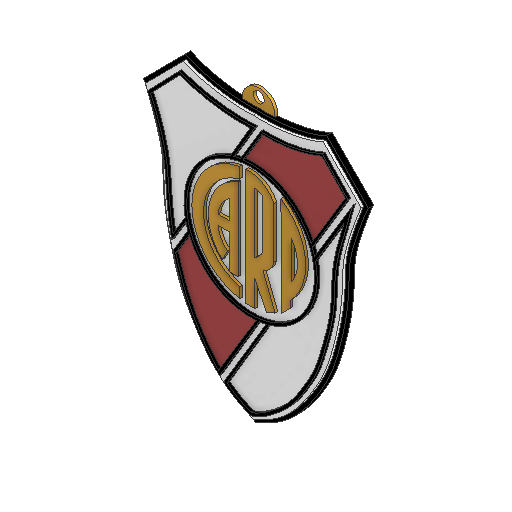
# Autodesk Inventor part: Sports Team Keychain
Saved by Autodesk Inventor 2026.2 (Build 302298000, 298)
## iProperties
Created: 2025-12-23
Part Number: Sports Team Keychain
Material: Generic
Document SubType Name: Modeling
Designer: andyeske
Density: 1 g/cm^3
Appearance: Default
Author: andyeske
Autodesk Inventor part; units mm, degrees
ref_plane "YZ Plane" through (0, 0, 0) normal (1, 0, 0) x (0, 1, 0)
ref_plane "XZ Plane" through (0, 0, 0) normal (0, 1, 0) x (-1, 0, 0)
ref_plane "XY Plane" through (0, 0, 0) normal (0, 0, 1) x (1, 0, 0)
sketch "Sketch1" plane through (0, 0, 0) normal (0, 0, 1) x (1, 0, 0)
  line L0 (-132.0665, 124.8918) -> (132.5169, 124.8918) construction
  line L1 (132.5169, 124.8918) -> (132.5169, -139.6916) construction
  line L2 (132.5169, -139.6916) -> (-132.0665, -139.6916) construction
  line L3 (-132.0665, -139.6916) -> (-132.0665, 124.8918) construction
  line L4 (0.2252, 52.8739) -> (0.2252, -73.7577) construction
  spline S0 degree 3 poles (0.2252, 52.8739) (-7.1403, 52.2049) (-23.4624, 53.7737) (-32.7052, 58.8275) knots 0 0 0 0 1 1 1 1
  line L5 (-32.7052, 58.8275) -> (-52.252, 39.1099)
  spline S1 degree 4 poles (-52.252, 39.1099) (-50.7995, 37.3406) (-43.3506, 15.7132) (-43.2795, 13.9138) (-43.0599, -7.6539) (-38.1267, -26.9843) (-33.574, -42.7818) (-15.201, -69.3664) (-7.1707, -69.2086) (0.2252, -73.7577) knots 0 0 0 0 0 0.249108 0.356574 0.465638 0.590869 0.717378 1 1 1 1 1
  spline S2 degree 3 poles (0.2252, 52.8739) (7.5907, 52.2049) (23.9128, 53.7737) (33.1557, 58.8275) knots 0 0 0 0 1 1 1 1
  line L6 (33.1557, 58.8275) -> (52.7024, 39.1099)
  spline S3 degree 4 poles (52.7024, 39.1099) (51.2499, 37.3406) (43.801, 15.7132) (43.7299, 13.9138) (43.5103, -7.6539) (38.5771, -26.9843) (34.0244, -42.7818) (15.6514, -69.3664) (7.6211, -69.2086) (0.2252, -73.7577) knots 0 0 0 0 0 0.249108 0.356574 0.465638 0.590869 0.717378 1 1 1 1 1
  line L7 (50.2121, 38.7692) -> (32.7643, 56.3696)
  line L8 (32.8267, 56.7373) -> (50.5783, 38.8306)
  line L9 (-50.1278, 38.8306) -> (-32.3763, 56.7373)
  circle A0 centre (0.2252, 1.113) radius 31.0921
  circle A1 centre (0.2252, 1.113) radius 29.8304
  arc A2 (-4.9144, 28.5122) -> (-4.8155, -24.875) centre (-0.0222, 1.8276) ccw
  arc A3 (-4.9144, 23.4163) -> (-4.8155, -20.0306) centre (0.7097, 1.7055) ccw
  arc A4 (-5.5588, 21.892) -> (-12.9917, -13.1761) centre (1.5498, 2.0635) ccw
  arc A5 (-9.6705, 13.2195) -> (-14.9692, 4.2431) centre (-2.5392, 2.9579) ccw
  arc A6 (-14.9692, -0.3288) -> (-10.4952, -8.5226) centre (-2.4753, 1.1746) ccw
  line L10 (-14.9692, -0.3288) -> (-9.6705, -0.3288)
  line L11 (-9.6705, -0.3288) -> (-9.6705, -16.3707)
  line L12 (-9.6705, -16.3707) -> (-5.5588, -16.3707)
  line L13 (-5.5588, -16.3707) -> (-5.5588, 21.892)
  line L14 (-9.6705, 13.2195) -> (-9.6705, 4.2431)
  line L15 (-9.6705, 4.2431) -> (-14.9692, 4.2431)
  line L16 (-10.4952, -8.5226) -> (-12.9917, -13.1761)
  line L17 (-4.8155, -20.0306) -> (-4.8155, -24.875)
  line L18 (-4.9144, 28.5122) -> (-4.9144, 23.4163)
  line L19 (-2.0198, 28.8256) -> (-2.0198, -25.345)
  line L20 (-2.0198, -25.345) -> (2.2612, -25.345)
  line L21 (2.2612, -25.345) -> (2.2612, -13.1046)
  line L22 (2.2612, -13.1046) -> (7.5833, -24.2139)
  line L23 (7.5833, -24.2139) -> (11.6912, -22.4528)
  line L24 (11.6912, -22.4528) -> (5.9834, -8.1423)
  line L25 (18.7175, -13.8348) -> (18.7175, -16.995)
  line L26 (18.7175, -16.995) -> (14.6967, -21.051)
  line L27 (14.6967, -21.051) -> (14.3943, 25.0785)
  line L28 (19.2337, -6.0507) -> (19.2337, 11.4074)
  line L29 (2.2612, 23.4163) -> (2.2612, -4.7023)
  line L30 (5.9834, -0.3288) -> (5.9834, 21.892)
  line L31 (11.1353, 21.5624) -> (11.1353, -2.0971)
  arc A7 (5.9834, 21.892) -> (2.2612, 23.4163) centre (1.1977, 15.5123) ccw
  arc A8 (11.1353, 21.5624) -> (-2.0198, 28.8256) centre (-0.5221, 15.9934) ccw
  arc A9 (2.2612, -4.7023) -> (5.9834, -0.3288) centre (-1.54, 2.3034) ccw
  arc A10 (5.9834, -8.1423) -> (11.1353, -2.0971) centre (2.8946, -0.2921) ccw
  arc A11 (19.2337, -6.0507) -> (19.2337, 11.4074) centre (7.6722, 2.6784) ccw
  arc A12 (18.7175, -13.8348) -> (14.3943, 25.0785) centre (0.6922, 3.8595) ccw
  arc A13 (-33.199, 52.8738) -> (2.2612, 47.7839) centre (-3.3286, 134.908) ccw
  line L32 (-33.199, 52.8738) -> (-47.9375, 37.5085)
  spline S4 degree 4 poles (-47.9375, 37.5085) (-46.8652, 36.0211) (-37.463, 13.2639) (-40.1687, 6.2328) (-38.1633, -9.6174) (-36.5654, -16.995) knots 0 0 0 0 0 0.485566 1 1 1 1 1
  line L33 (-46.4307, 37.3236) -> (-32.8677, 51.4634)
  arc A14 (-32.8677, 51.4634) -> (0, 46.4519) centre (-3.3286, 134.908) ccw
  line L34 (-35.9295, -14.0185) -> (-30.2885, -4.8559)
  line L35 (-36.5654, -16.995) -> (-29.9733, -6.2874)
  line L36 (2.2612, 47.7839) -> (-7.614, 31.2006)
  line L37 (-9.2032, 30.7411) -> (0, 46.4519)
  arc A15 (4.9226, 47.558) -> (33.6498, 52.8624) centre (7.7691, 112.5842) ccw
  line L38 (33.6498, 52.8624) -> (45.6523, 40.3328)
  arc A16 (5.5282, 46.6286) -> (33.4296, 51.7837) centre (7.7691, 112.5842) ccw
  line L39 (33.4296, 51.7837) -> (44.4012, 40.3303)
  line L40 (4.9226, 47.558) -> (-4.6016, 31.8281)
  line L41 (-3.3284, 32.0013) -> (5.5282, 46.6286)
  line L42 (45.6523, 40.3328) -> (29.0153, 12.8539)
  line L43 (28.4601, 14.1326) -> (44.4012, 40.3303)
  spline S5 degree 4 poles (48.0149, 39.324) (46.5349, 35.8952) (45.4135, 28.3855) (41.1447, 18.7455) (39.3482, 4.364) (39.4943, -4.0682) (38.3845, -14.3456) (33.0006, -32.0454) (31.1325, -37.6554) (22.582, -52.5964) (16.6222, -60.5054) (4.0219, -69.3118) (0.2252, -69.5232) knots 0 0 0 0 0 0.185243 0.265386 0.348089 0.436947 0.523089 0.611425 0.699576 0.784821 1 1 1 1 1
  spline S6 degree 2 poles (-12.3198, -62.2786) (-7.9831, -66.4046) (0.2252, -69.5232) knots 0 0 0 1 1 1
  line L44 (-12.3198, -62.2786) -> (7.4298, -29.1329)
  line L45 (8.8369, -28.7627) -> (-10.7246, -61.848)
  line L46 (30.128, 9.6301) -> (48.0149, 39.324)
  line L47 (30.5524, 7.9672) -> (43.7735, 29.8042)
  spline S7 degree 4 poles (-35.9289, -21.0539) (-32.599, -31.9567) (-30.1057, -43.8341) (-16.8017, -59.2056) (-14.1645, -60.568) knots 0 0 0 0 0 1 1 1 1 1
  line L48 (-35.9289, -21.0539) -> (-29.0211, -9.4401)
  line L49 (-14.1645, -60.568) -> (4.1798, -29.7266)
  line L50 (2.7836, -29.8736) -> (-14.6898, -58.73)
  line L51 (-28.4185, -10.9806) -> (-34.7089, -21.1968)
  spline S8 degree 5 poles (-32.3763, 56.7373) (-30.9924, 56.0576) (-29.5669, 55.4625) (-28.1175, 54.9329) (-24.8224, 53.8685) (-21.4582, 53.0455) (-19.5794, 52.65) (-15.9119, 51.9875) (-12.2148, 51.5192) (-10.4169, 51.3356) (-7.2106, 51.0872) (-3.996, 51.0024) (-2.5875, 51.003) (-1.1779, 51.0424) (0.2252, 51.1622) knots 0 0 0 0 0 0 0.230969 0.230969 0.230969 0.518425 0.518425 0.518425 0.789049 0.789049 0.789049 1 1 1 1 1 1
  spline S9 degree 5 poles (0.2252, 51.1622) (1.6284, 51.0424) (3.0379, 51.003) (4.4464, 51.0024) (7.661, 51.0872) (10.8673, 51.3356) (12.6652, 51.5192) (16.3623, 51.9875) (20.0299, 52.65) (21.9086, 53.0455) (25.2729, 53.8685) (28.5679, 54.9329) (30.0174, 55.4625) (31.4428, 56.0576) (32.8267, 56.7373) knots 0 0 0 0 0 0 0.210951 0.210951 0.210951 0.481575 0.481575 0.481575 0.769031 0.769031 0.769031 1 1 1 1 1 1
  spline S10 degree 5 poles (50.5784, 38.8305) (50.4716, 38.6118) (50.3681, 38.3916) (50.2669, 38.1704) (49.8396, 37.2091) (49.4397, 36.2373) (49.1407, 35.4861) (48.5055, 33.852) (47.8955, 32.2077) (47.5719, 31.3194) (46.9324, 29.5307) (46.3128, 27.7351) (46.0067, 26.8314) (45.4296, 25.095) (44.8751, 23.3512) (44.6155, 22.5147) (44.1437, 20.95) (43.7022, 19.3765) (43.505, 18.6441) (43.1571, 17.2809) (42.8515, 15.9077) (42.7212, 15.2725) (42.4981, 14.0593) (42.3266, 12.8377) (42.2579, 12.2566) (42.1442, 11.0801) (42.0717, 9.9003) (42.0433, 9.3042) (41.9937, 8.0313) (41.9583, 6.7579) (41.9404, 6.0811) (41.8996, 4.6148) (41.849, 3.1488) (41.817, 2.3596) (41.7369, 0.6804) (41.6275, -0.9972) (41.5599, -1.886) (41.3991, -3.7303) (41.1949, -5.5702) (41.0773, -6.5229) (40.8142, -8.4577) (40.5048, -10.3856) (40.3359, -11.3638) (39.9774, -13.3105) (39.5793, -15.2494) (39.3718, -16.2141) (38.9517, -18.0968) (38.5051, -19.9735) (38.2811, -20.8888) (37.8369, -22.6557) (37.37, -24.4168) (37.1389, -25.2654) (36.6778, -26.9096) (36.1881, -28.5454) (35.9429, -29.3363) (35.4363, -30.9056) (34.8885, -32.4609) (34.6042, -33.2312) (33.9913, -34.8132) (33.3272, -36.3745) (32.971, -37.1744) (32.1969, -38.8428) (31.372, -40.4867) (30.9271, -41.3415) (29.9757, -43.1097) (28.9768, -44.8516) (28.4455, -45.7507) (27.3422, -47.5647) (26.1925, -49.3496) (25.5965, -50.2489) (24.3957, -52.0079) (23.1449, -53.7316) (22.5149, -54.5728) (21.2732, -56.1759) (19.977, -57.7352) (19.339, -58.475) (18.0987, -59.8565) (16.8013, -61.1844) (16.1728, -61.8001) (14.9573, -62.9344) (13.6867, -64.0064) (13.0757, -64.4959) (11.8869, -65.3962) (10.6518, -66.2317) (10.0549, -66.6134) (8.8698, -67.3295) (7.6544, -67.9927) (7.0548, -68.3053) (5.829, -68.9226) (4.5933, -69.5198) (3.9658, -69.8216) (2.8318, -70.375) (1.7096, -70.9521) (1.2101, -71.2174) (0.7151, -71.4909) (0.2252, -71.7733) knots 0 0 0 0 0 0 0.009552 0.009552 0.009552 0.041262 0.041262 0.041262 0.078369 0.078369 0.078369 0.11581 0.11581 0.11581 0.15018 0.15018 0.15018 0.179945 0.179945 0.179945 0.205387 0.205387 0.205387 0.228345 0.228345 0.228345 0.251767 0.251767 0.251767 0.278338 0.278338 0.278338 0.309334 0.309334 0.309334 0.344313 0.344313 0.344313 0.381983 0.381983 0.381983 0.420938 0.420938 0.420938 0.459661 0.459661 0.459661 0.496643 0.496643 0.496643 0.53116 0.53116 0.53116 0.563654 0.563654 0.563654 0.595872 0.595872 0.595872 0.63023 0.63023 0.63023 0.668044 0.668044 0.668044 0.709026 0.709026 0.709026 0.751362 0.751362 0.751362 0.792601 0.792601 0.792601 0.830929 0.830929 0.830929 0.865445 0.865445 0.865445 0.896154 0.896154 0.896154 0.923948 0.923948 0.923948 0.95048 0.95048 0.95048 0.977808 0.977808 0.977808 1 1 1 1 1 1
  spline S11 degree 5 poles (0.2252, -71.7733) (-0.2646, -71.4909) (-0.7597, -71.2174) (-1.2591, -70.9521) (-2.3813, -70.375) (-3.5154, -69.8216) (-4.1429, -69.5198) (-5.3786, -68.9226) (-6.6044, -68.3053) (-7.2039, -67.9927) (-8.4193, -67.3295) (-9.6044, -66.6134) (-10.2014, -66.2317) (-11.4364, -65.3962) (-12.6253, -64.4959) (-13.2363, -64.0064) (-14.5069, -62.9344) (-15.7224, -61.8001) (-16.3509, -61.1844) (-17.6483, -59.8565) (-18.8886, -58.475) (-19.5265, -57.7352) (-20.8228, -56.1759) (-22.0645, -54.5728) (-22.6945, -53.7316) (-23.9453, -52.0079) (-25.1461, -50.2489) (-25.7421, -49.3496) (-26.8917, -47.5647) (-27.995, -45.7507) (-28.5264, -44.8516) (-29.5252, -43.1097) (-30.4767, -41.3415) (-30.9216, -40.4867) (-31.7465, -38.8428) (-32.5206, -37.1744) (-32.8767, -36.3745) (-33.5408, -34.8132) (-34.1538, -33.2312) (-34.4381, -32.4609) (-34.9859, -30.9056) (-35.4925, -29.3363) (-35.7377, -28.5454) (-36.2274, -26.9096) (-36.6884, -25.2654) (-36.9195, -24.4168) (-37.3865, -22.6557) (-37.8306, -20.8888) (-38.0546, -19.9735) (-38.5013, -18.0968) (-38.9214, -16.2141) (-39.1288, -15.2494) (-39.527, -13.3105) (-39.8855, -11.3638) (-40.0544, -10.3856) (-40.3638, -8.4577) (-40.6268, -6.5229) (-40.7445, -5.5702) (-40.9487, -3.7303) (-41.1095, -1.886) (-41.1771, -0.9972) (-41.2865, 0.6804) (-41.3666, 2.3596) (-41.3985, 3.1488) (-41.4492, 4.6148) (-41.49, 6.0811) (-41.5079, 6.7579) (-41.5433, 8.0313) (-41.5929, 9.3042) (-41.6212, 9.9003) (-41.6938, 11.0801) (-41.8075, 12.2566) (-41.8761, 12.8377) (-42.0476, 14.0593) (-42.2708, 15.2725) (-42.4011, 15.9077) (-42.7067, 17.2809) (-43.0546, 18.6441) (-43.2517, 19.3765) (-43.6933, 20.95) (-44.165, 22.5147) (-44.4247, 23.3512) (-44.9792, 25.095) (-45.5563, 26.8314) (-45.8624, 27.7351) (-46.4819, 29.5307) (-47.1215, 31.3194) (-47.445, 32.2077) (-48.055, 33.852) (-48.6903, 35.4861) (-48.9892, 36.2373) (-49.3892, 37.2091) (-49.8165, 38.1704) (-49.9177, 38.3916) (-50.0212, 38.6118) (-50.128, 38.8305) knots 0 0 0 0 0 0 0.022192 0.022192 0.022192 0.04952 0.04952 0.04952 0.076052 0.076052 0.076052 0.103846 0.103846 0.103846 0.134555 0.134555 0.134555 0.169071 0.169071 0.169071 0.207399 0.207399 0.207399 0.248638 0.248638 0.248638 0.290974 0.290974 0.290974 0.331956 0.331956 0.331956 0.36977 0.36977 0.36977 0.404128 0.404128 0.404128 0.436346 0.436346 0.436346 0.46884 0.46884 0.46884 0.503357 0.503357 0.503357 0.540339 0.540339 0.540339 0.579062 0.579062 0.579062 0.618017 0.618017 0.618017 0.655687 0.655687 0.655687 0.690666 0.690666 0.690666 0.721662 0.721662 0.721662 0.748233 0.748233 0.748233 0.771655 0.771655 0.771655 0.794613 0.794613 0.794613 0.820055 0.820055 0.820055 0.84982 0.84982 0.84982 0.88419 0.88419 0.88419 0.921631 0.921631 0.921631 0.958738 0.958738 0.958738 0.990448 0.990448 0.990448 1 1 1 1 1 1
  spline S12 degree 5 poles (-35.9295, -14.0185) (-35.9545, -13.8865) (-35.9794, -13.7544) (-36.004, -13.6223) (-36.1541, -12.8108) (-36.2967, -11.998) (-36.4107, -11.3166) (-36.6265, -9.9642) (-36.8219, -8.6087) (-36.9137, -7.9362) (-37.0851, -6.6099) (-37.2377, -5.2814) (-37.3085, -4.6265) (-37.4393, -3.3382) (-37.5547, -2.0484) (-37.608, -1.4143) (-37.7067, -0.1645) (-37.7955, 1.086) (-37.8372, 1.702) (-37.9173, 2.9236) (-37.9951, 4.1453) (-38.0338, 4.751) (-38.1136, 5.9655) (-38.2014, 7.1794) (-38.2483, 7.7878) (-38.352, 9.0261) (-38.4758, 10.2625) (-38.545, 10.8912) (-38.7026, 12.1898) (-38.8923, 13.4842) (-38.9993, 14.1515) (-39.2404, 15.5369) (-39.5184, 16.9155) (-39.6725, 17.6296) (-40.0096, 19.1029) (-40.3827, 20.5676) (-40.5843, 21.3221) (-41.0117, 22.8545) (-41.4711, 24.3776) (-41.7127, 25.1507) (-42.2072, 26.6821) (-42.7291, 28.2044) (-42.9948, 28.9583) (-43.5158, 30.397) (-44.0606, 31.8269) (-44.3266, 32.5076) (-44.8166, 33.732) (-45.3298, 34.9466) (-45.5635, 35.4863) (-45.8736, 36.179) (-46.2009, 36.8642) (-46.2761, 37.018) (-46.3525, 37.1712) (-46.4307, 37.3235) knots 0 0 0 0 0 0 0.012737 0.012737 0.012737 0.078207 0.078207 0.078207 0.142524 0.142524 0.142524 0.204941 0.204941 0.204941 0.265247 0.265247 0.265247 0.323751 0.323751 0.323751 0.381267 0.381267 0.381267 0.439097 0.439097 0.439097 0.499027 0.499027 0.499027 0.563065 0.563065 0.563065 0.632289 0.632289 0.632289 0.706295 0.706295 0.706295 0.78305 0.78305 0.78305 0.8588 0.8588 0.8588 0.928059 0.928059 0.928059 0.983771 0.983771 0.983771 1 1 1 1 1 1
  spline S13 degree 5 poles (-10.7246, -61.848) (-8.7925, -63.5382) (-6.609, -64.9388) (-4.3337, -66.1331) (-1.9832, -67.1787) (0.4116, -68.1026) knots 0 0 0 0 0 0 1 1 1 1 1 1
  spline S14 degree 5 poles (0.4116, -68.1025) (0.7622, -68.0477) (1.1058, -67.9475) (1.4427, -67.8385) (2.3734, -67.4856) (3.2714, -67.0579) (3.8394, -66.7638) (5.0604, -66.0907) (6.2473, -65.3582) (6.8815, -64.9484) (8.1683, -64.0815) (9.423, -63.1688) (10.0589, -62.6894) (11.3072, -61.7152) (12.5227, -60.7002) (13.1186, -60.1858) (14.2653, -59.1615) (15.3762, -58.0985) (15.9094, -57.5704) (16.9271, -56.5249) (17.9059, -55.4429) (18.3715, -54.9088) (19.267, -53.8417) (20.1232, -52.7429) (20.5344, -52.1957) (21.3431, -51.0826) (22.1197, -49.9469) (22.5028, -49.3713) (23.2668, -48.1967) (24.0087, -47.008) (24.3797, -46.4029) (25.111, -45.1908) (25.8261, -43.9691) (26.1788, -43.3576) (26.8512, -42.1745) (27.5063, -40.9817) (27.8171, -40.4051) (28.3943, -39.3096) (28.9472, -38.2016) (29.2012, -37.6766) (29.6804, -36.6479) (30.1269, -35.6047) (30.3354, -35.0942) (30.7594, -34.0059) (31.1521, -32.906) (31.3526, -32.3231) (31.7882, -31.0215) (32.205, -29.7137) (32.4309, -28.9921) (32.9165, -27.417) (33.3892, -25.8379) (33.6418, -24.9822) (34.1558, -23.2148) (34.6528, -21.4425) (34.9036, -20.5277) (35.3804, -18.7405) (35.8284, -16.9459) (36.0388, -16.0696) (36.4178, -14.4144) (36.7579, -12.7508) (36.9077, -11.9681) (37.1668, -10.5007) (37.3828, -9.0264) (37.4733, -8.3391) (37.6265, -7.0275) (37.7444, -5.7124) (37.7927, -5.0871) (37.8737, -3.8625) (37.9331, -2.6366) (37.958, -2.0371) (38.003, -0.8304) (38.0436, 0.3765) (38.0644, 0.9836) (38.1117, 2.2301) (38.1721, 3.4761) (38.2079, 4.115) (38.2931, 5.4326) (38.4038, 6.7483) (38.4683, 7.4257) (38.6158, 8.8094) (38.7966, 10.1891) (38.8979, 10.8929) (39.1207, 12.3059) (39.3818, 13.7124) (39.5229, 14.418) (39.8223, 15.8153) (40.1575, 17.2045) (40.3323, 17.8921) (40.6919, 19.2446) (41.0751, 20.5905) (41.2685, 21.2528) (41.6544, 22.5558) (42.0454, 23.8574) (42.238, 24.4982) (42.6152, 25.7604) (42.9861, 27.0245) (43.1666, 27.6471) (43.3964, 28.4521) (43.622, 29.2582) (43.6727, 29.4402) (43.7232, 29.6221) (43.7735, 29.8042) knots 0 0 0 0 0 0 0.015802 0.015802 0.015802 0.044244 0.044244 0.044244 0.07785 0.07785 0.07785 0.113289 0.113289 0.113289 0.148321 0.148321 0.148321 0.181716 0.181716 0.181716 0.213249 0.213249 0.213249 0.243707 0.243707 0.243707 0.274481 0.274481 0.274481 0.30607 0.30607 0.30607 0.337488 0.337488 0.337488 0.366639 0.366639 0.366639 0.392599 0.392599 0.392599 0.41714 0.41714 0.41714 0.444576 0.444576 0.444576 0.47823 0.47823 0.47823 0.517941 0.517941 0.517941 0.560156 0.560156 0.560156 0.600266 0.600266 0.600266 0.635729 0.635729 0.635729 0.666581 0.666581 0.666581 0.694495 0.694495 0.694495 0.721203 0.721203 0.721203 0.748243 0.748243 0.748243 0.776723 0.776723 0.776723 0.807009 0.807009 0.807009 0.838653 0.838653 0.838653 0.870673 0.870673 0.870673 0.902252 0.902252 0.902252 0.932959 0.932959 0.932959 0.962741 0.962741 0.962741 0.991594 0.991594 0.991594 1 1 1 1 1 1
  spline S15 degree 5 poles (-34.7089, -21.1968) (-34.5806, -21.6211) (-34.4534, -22.0458) (-34.327, -22.4708) (-34.0446, -23.4218) (-33.7619, -24.3728) (-33.6047, -24.8986) (-33.2842, -25.9597) (-32.9558, -27.0184) (-32.7874, -27.5522) (-32.4405, -28.6307) (-32.0799, -29.7047) (-31.8937, -30.2468) (-31.508, -31.3422) (-31.1046, -32.4312) (-30.8957, -32.9808) (-30.4628, -34.0899) (-30.0098, -35.1909) (-29.7752, -35.7459) (-29.2907, -36.8629) (-28.7847, -37.9704) (-28.5236, -38.5273) (-27.9868, -39.6439) (-27.4283, -40.7498) (-27.1416, -41.3039) (-26.556, -42.4091) (-25.9491, -43.5027) (-25.6396, -44.0479) (-25.0126, -45.1283) (-24.3652, -46.1966) (-24.0378, -46.7257) (-23.3807, -47.7654) (-22.7045, -48.7928) (-22.3657, -49.2973) (-21.694, -50.278) (-21.0044, -51.2462) (-20.6631, -51.7164) (-19.9962, -52.6174) (-19.3127, -53.5058) (-18.9795, -53.9307) (-18.3412, -54.7288) (-17.6872, -55.5141) (-17.3751, -55.8814) (-16.794, -56.5505) (-16.1978, -57.2061) (-15.9223, -57.5018) (-15.5142, -57.9288) (-15.0949, -58.3446) (-14.9614, -58.4747) (-14.8265, -58.6033) (-14.6898, -58.73) knots 0 0 0 0 0 0 0.051523 0.051523 0.051523 0.1153 0.1153 0.1153 0.180345 0.180345 0.180345 0.246965 0.246965 0.246965 0.315302 0.315302 0.315302 0.385323 0.385323 0.385323 0.456801 0.456801 0.456801 0.5293 0.5293 0.5293 0.602155 0.602155 0.602155 0.674467 0.674467 0.674467 0.745087 0.745087 0.745087 0.812608 0.812608 0.812608 0.875356 0.875356 0.875356 0.93137 0.93137 0.93137 0.97834 0.97834 0.97834 1 1 1 1 1 1
  point P0 (0, 0)
  point P1 (-7.8471, 52.8738)
  point P2 (-21.0342, 54.7365)
  point P3 (-47.9375, 28.5118)
  point P4 (-43.9836, 15.1044)
  point P5 (-43.2605, 8.251)
  point P6 (-42.4783, -5.362)
  point P7 (-38.5204, -25.0154)
  point P8 (-33.199, -39.7232)
  point P9 (-20.5679, -59.1245)
  point P10 (-9.204, -68.8277)
  point P11 (8.2975, 52.8738)
  point P12 (21.4846, 54.7365)
  point P13 (48.3879, 28.5118)
  point P14 (44.434, 15.1044)
  point P15 (43.711, 8.251)
  point P16 (42.9287, -5.362)
  point P17 (38.9708, -25.0154)
  point P18 (33.6495, -39.7232)
  point P19 (21.0183, -59.1245)
  point P20 (9.6544, -68.8277)
  point P21 (-45.0314, 30.9544)
  point P22 (-40.575, 15.9863)
  point P23 (-39.3069, 5.5697)
  point P24 (-38.5202, -4.7019)
  point P25 (46.2203, 33.5463)
  point P26 (43.8649, 25.0795)
  point P27 (41.1003, 15.1053)
  point P28 (39.6519, 4.8092)
  point P29 (39.2858, -3.4591)
  point P30 (37.7873, -14.6267)
  point P31 (33.1555, -31.3065)
  point P32 (30.2746, -38.6482)
  point P33 (25.2393, -47.6606)
  point P34 (18.7174, -56.615)
  point P35 (8.2976, -65.6679)
  point P36 (-7.6169, -65.7976)
  point P37 (-31.7692, -33.8334)
  point P38 (-24.2495, -48.4847)
  point P39 (-16.672, -58.3427)
  constraints: 97 end point, 32 point on circle, 16 centre point, 12 symmetric about line, 9 parallel, 8 vertical, 5 perpendicular, 3 point on line, 2 horizontal, 106 other
sketch "Sketch2" plane through (0, 0, 0) normal (0, 0, 1) x (1, 0, 0)
  line L0 (-32.7052, 58.8275) -> (-52.252, 39.1099) projected
  spline S0 degree 3 poles (0.2252, 52.8739) (-7.1403, 52.2049) (-23.4624, 53.7737) (-32.7052, 58.8275) knots 0 0 0 0 1 1 1 1 projected
  spline S1 degree 3 poles (0.2252, 52.8739) (7.5907, 52.2049) (23.9128, 53.7737) (33.1557, 58.8275) knots 0 0 0 0 1 1 1 1 projected
  line L1 (33.1557, 58.8275) -> (52.7024, 39.1099) projected
  spline S2 degree 4 poles (52.7024, 39.1099) (51.2499, 37.3406) (43.801, 15.7132) (43.7299, 13.9138) (43.5103, -7.6539) (38.5771, -26.9843) (34.0244, -42.7818) (15.6514, -69.3664) (7.6211, -69.2086) (0.2252, -73.7577) knots 0 0 0 0 0 0.249108 0.356574 0.465638 0.590869 0.717378 1 1 1 1 1 projected
  spline S3 degree 4 poles (-52.252, 39.1099) (-50.7995, 37.3406) (-43.3506, 15.7132) (-43.2795, 13.9138) (-43.0599, -7.6539) (-38.1267, -26.9843) (-33.574, -42.7818) (-15.201, -69.3664) (-7.1707, -69.2086) (0.2252, -73.7577) knots 0 0 0 0 0 0.249108 0.356574 0.465638 0.590869 0.717378 1 1 1 1 1 projected
  point P0 (0, 0)
extrude "Extrusion1" add sketch "Sketch2" along normal blind 2.54
sketch "Sketch3" plane through (0, 0, 2.54) normal (0, 0, 1) x (1, 0, 0)
  line L0 (4.9226, 47.558) -> (-4.6016, 31.8281) projected
  arc A0 (4.9226, 47.558) -> (33.6498, 52.8624) centre (7.7691, 112.5842) ccw projected
  line L1 (33.6498, 52.8624) -> (45.6523, 40.3328) projected
  line L2 (45.6523, 40.3328) -> (29.0153, 12.8539) projected
  circle A1 centre (0.2252, 1.113) radius 31.0921 projected
  line L3 (2.2612, 47.7839) -> (-7.614, 31.2006) projected
  arc A2 (-33.199, 52.8738) -> (2.2612, 47.7839) centre (-3.3286, 134.908) ccw projected
  line L4 (-33.199, 52.8738) -> (-47.9375, 37.5085) projected
  spline S0 degree 4 poles (-47.9375, 37.5085) (-46.8652, 36.0211) (-37.463, 13.2639) (-40.1687, 6.2328) (-38.1633, -9.6174) (-36.5654, -16.995) knots 0 0 0 0 0 0.485566 1 1 1 1 1 projected
  line L5 (-36.5654, -16.995) -> (-29.9733, -6.2874) projected
  line L6 (-35.9289, -21.0539) -> (-29.0211, -9.4401) projected
  spline S1 degree 4 poles (-35.9289, -21.0539) (-32.599, -31.9567) (-30.1057, -43.8341) (-16.8017, -59.2056) (-14.1645, -60.568) knots 0 0 0 0 0 1 1 1 1 1 projected
  line L7 (-14.1645, -60.568) -> (4.1798, -29.7266) projected
  line L8 (-12.3198, -62.2786) -> (7.4298, -29.1329) projected
  spline S2 degree 2 poles (-12.3198, -62.2786) (-7.9831, -66.4046) (0.2252, -69.5232) knots 0 0 0 1 1 1 projected
  spline S3 degree 4 poles (48.0149, 39.324) (46.5349, 35.8952) (45.4135, 28.3855) (41.1447, 18.7455) (39.3482, 4.364) (39.4943, -4.0682) (38.3845, -14.3456) (33.0006, -32.0454) (31.1325, -37.6554) (22.582, -52.5964) (16.6222, -60.5054) (4.0219, -69.3118) (0.2252, -69.5232) knots 0 0 0 0 0 0.185243 0.265386 0.348089 0.436947 0.523089 0.611425 0.699576 0.784821 1 1 1 1 1 projected
  line L9 (30.128, 9.6301) -> (48.0149, 39.324) projected
  line L10 (-3.3284, 32.0013) -> (5.5282, 46.6286) projected
  arc A3 (5.5282, 46.6286) -> (33.4296, 51.7837) centre (7.7691, 112.5842) ccw projected
  line L11 (33.4296, 51.7837) -> (44.4012, 40.3303) projected
  line L12 (28.4601, 14.1326) -> (44.4012, 40.3303) projected
  circle A4 centre (0.2252, 1.113) radius 29.8304 projected
  line L13 (-9.2032, 30.7411) -> (0, 46.4519) projected
  arc A5 (-32.8677, 51.4634) -> (0, 46.4519) centre (-3.3286, 134.908) ccw projected
  spline S4 degree 3 poles (-35.9295, -14.0185) (-36.2087, -12.5467) (-36.6458, -9.9525) (-37.0338, -7.0433) (-37.2803, -4.9008) (-37.4236, -3.4937) (-37.5799, -1.7629) (-37.6884, -0.4004) (-37.8092, 1.2782) (-37.8964, 2.6035) (-38.0015, 4.2459) (-38.0859, 5.5524) (-38.2015, 7.1877) (-38.3065, 8.5034) (-38.4652, 10.1725) (-38.6196, 11.5344) (-38.8606, 13.2879) (-39.0967, 14.7368) (-39.4534, 16.6115) (-39.7898, 18.1623) (-40.2261, 19.9589) (-40.5483, 21.1824) (-40.8938, 22.4211) (-41.1354, 23.2534) (-41.4502, 24.2986) (-41.7116, 25.1372) (-42.0489, 26.1846) (-42.3263, 27.02) (-42.7512, 28.2634) (-43.1861, 29.4898) (-43.8455, 31.2711) (-44.4297, 32.7716) (-45.0608, 34.3137) (-45.4595, 35.2444) (-45.8314, 36.0774) (-46.1226, 36.7062) (-46.3321, 37.1315) (-46.4307, 37.3236) knots 0.036168 0.036168 0.036168 0.036168 0.112537 0.169813 0.188906 0.22709 0.246182 0.284366 0.303458 0.341643 0.360735 0.398919 0.418011 0.456195 0.475287 0.513472 0.532564 0.570748 0.58984 0.628024 0.647117 0.675755 0.685301 0.704393 0.713939 0.733031 0.742577 0.761669 0.771215 0.799854 0.818946 0.85713 0.876222 0.90486 0.914406 0.933499 0.952591 0.952591 0.952591 0.952591 projected
  line L14 (-35.9295, -14.0185) -> (-30.2885, -4.8559) projected
  line L15 (-28.4185, -10.9806) -> (-34.7089, -21.1968) projected
  spline S5 degree 3 poles (-34.7089, -21.1968) (-34.3745, -22.3027) (-33.8033, -24.2491) (-33.117, -26.5097) (-32.5728, -28.2225) (-32.1931, -29.3732) (-31.6928, -30.8223) (-31.2704, -31.9899) (-30.7116, -33.4585) (-30.2389, -34.6399) (-29.6145, -36.1226) (-29.0877, -37.3123) (-28.3949, -38.8006) (-27.8136, -39.9906) (-27.0544, -41.473) (-26.4219, -42.6528) (-25.6027, -44.1148) (-24.9261, -45.2716) (-24.058, -46.6956) (-23.3478, -47.8142) (-22.4465, -49.1797) (-21.7173, -50.2427) (-20.8031, -51.5263) (-20.073, -52.5137) (-19.171, -53.6891) (-18.462, -54.5786) (-17.6024, -55.6163) (-16.9408, -56.3829) (-16.1593, -57.2498) (-15.4304, -58.0192) (-14.9206, -58.5159) (-14.6898, -58.73) knots 0.010734 0.010734 0.010734 0.010734 0.086163 0.142734 0.161591 0.199305 0.218162 0.255877 0.274734 0.312448 0.331305 0.36902 0.387877 0.425591 0.444448 0.482162 0.501019 0.538734 0.557591 0.595305 0.614162 0.651876 0.670734 0.708448 0.727305 0.765019 0.783876 0.821591 0.840448 0.878162 0.915876 0.915876 0.915876 0.915876 projected
  line L16 (2.7836, -29.8736) -> (-14.6898, -58.73) projected
  line L17 (8.8369, -28.7627) -> (-10.7246, -61.848) projected
  spline S6 degree 3 poles (-10.7246, -61.848) (-10.506, -62.0392) (-10.0538, -62.4191) (-9.451, -62.8874) (-8.8199, -63.3505) (-8.2923, -63.7168) (-7.6043, -64.1692) (-7.0313, -64.5268) (-6.2864, -64.968) (-5.6678, -65.3165) (-4.8661, -65.7461) (-4.2019, -66.085) (-3.3432, -66.5026) (-2.6335, -66.8318) (-1.718, -67.237) (-0.7741, -67.6359) (0.0113, -67.9481) (0.4116, -68.1026) knots 0.075596 0.075596 0.075596 0.075596 0.151022 0.226449 0.264162 0.339589 0.377302 0.452728 0.490442 0.565868 0.603582 0.679008 0.716721 0.792148 0.829861 0.905288 0.980714 0.980714 0.980714 0.980714 projected
  spline S7 degree 3 poles (0.4116, -68.1026) (0.5829, -68.0755) (0.9926, -67.9833) (1.6226, -67.771) (2.3176, -67.4925) (2.9187, -67.2198) (3.7117, -66.8241) (4.3747, -66.4667) (5.2287, -65.976) (5.9285, -65.5509) (6.8155, -64.9852) (7.5321, -64.5073) (8.4298, -63.8838) (9.1471, -63.366) (10.0372, -62.6996) (10.7421, -62.1528) (11.6099, -61.456) (12.292, -60.8893) (13.1262, -60.1723) (13.7777, -59.5929) (14.5702, -58.8635) (15.1859, -58.2767) (15.9317, -57.5405) (16.509, -56.9497) (17.2065, -56.2096) (17.7452, -55.6162) (18.3957, -54.8728) (18.8983, -54.2763) (19.628, -53.3777) (20.3276, -52.4725) (21.2225, -51.2463) (21.8739, -50.3062) (22.5156, -49.3468) (22.9394, -48.6976) (23.4651, -47.8744) (23.8828, -47.2071) (24.4013, -46.3638) (24.8128, -45.683) (25.3218, -44.8276) (25.724, -44.1414) (26.2178, -43.2861) (26.6044, -42.6059) (27.0735, -41.7671) (27.4358, -41.1074) (27.87, -40.3007) (28.2016, -39.6707) (28.5954, -38.9031) (28.8936, -38.3047) (29.2462, -37.5739) (29.5127, -37.0014) (29.8285, -36.2952) (30.0687, -35.7347) (30.3573, -35.0302) (30.5809, -34.4592) (30.8566, -33.7234) (31.0767, -33.1115) (31.3562, -32.3066) (31.5846, -31.6274) (31.8793, -30.7284) (32.123, -29.9676) (32.4386, -28.9633) (32.7, -28.1173) (33.0371, -27.0093) (33.3145, -26.0845) (33.6681, -24.8875) (33.9553, -23.9005) (34.3152, -22.6414) (34.6017, -21.6195) (34.9524, -20.3377) (35.2251, -19.3136) (35.552, -18.0463) (35.8007, -17.0465) (36.0929, -15.8222) (36.3106, -14.8657) (36.5612, -13.7037) (36.7439, -12.8023) (36.95, -11.7127) (37.097, -10.8707) (37.2921, -9.6504) (37.4545, -8.4843) (37.6469, -6.8162) (37.7703, -5.4057) (37.8824, -3.6982) (37.9452, -2.3629) (38.0076, -0.7004) (38.0516, 0.6365) (38.1107, 2.1733) (38.1597, 3.2208) (38.2206, 4.2901) (38.268, 5.014) (38.3369, 5.9329) (38.4004, 6.6791) (38.4914, 7.6248) (38.5739, 8.3911) (38.7131, 9.5527) (38.8736, 10.7286) (39.1563, 12.5052) (39.4528, 14.0862) (39.8336, 15.8488) (40.1115, 17.0112) (40.4052, 18.1604) (40.608, 18.9195) (40.9203, 20.0473) (41.2413, 21.16) (41.7285, 22.8034) (42.1611, 24.2408) (42.6893, 26.0118) (43.2008, 27.758) (43.5866, 29.1275) (43.7735, 29.8042) knots 0.102833 0.102833 0.102833 0.102833 0.112122 0.121411 0.126055 0.135344 0.139988 0.149277 0.153921 0.16321 0.167854 0.177143 0.181787 0.191076 0.195721 0.205009 0.209654 0.218942 0.223587 0.232876 0.23752 0.246809 0.251453 0.260742 0.265386 0.274675 0.279319 0.288608 0.293252 0.307186 0.316474 0.330407 0.335052 0.344341 0.348985 0.358274 0.362918 0.372207 0.376851 0.38614 0.390784 0.400073 0.404717 0.414006 0.418651 0.427939 0.432584 0.441872 0.446517 0.455806 0.46045 0.469739 0.474383 0.483672 0.488316 0.497605 0.502249 0.511538 0.516182 0.525471 0.530116 0.539404 0.544049 0.553337 0.557982 0.567271 0.571915 0.581204 0.585848 0.595137 0.599781 0.60907 0.613714 0.623003 0.627648 0.636936 0.641581 0.650869 0.655514 0.669447 0.678736 0.697313 0.706602 0.725179 0.734468 0.753046 0.762334 0.776268 0.780912 0.790201 0.794845 0.804134 0.808778 0.818067 0.822711 0.836644 0.845933 0.864511 0.873799 0.887733 0.892377 0.901666 0.90631 0.920243 0.929532 0.948109 0.957398 0.975976 0.994553 0.994553 0.994553 0.994553 projected
  line L18 (30.5524, 7.9672) -> (43.7735, 29.8042) projected
  line L19 (-46.4307, 37.3236) -> (-32.8677, 51.4634) projected
  point P0 (0, 0)
  constraints: 1 other
extrude "Extrusion2" add sketch "Sketch3" along normal blind 2.54 contours A0 L1 L2 A1 L12 L11 A3 L10 L0 | A1 | A1 L13 A5 L19 S4 L14 L5 S0 L4 A2 L3 | L9 S3 S2 L8 A1 L17 S6 S7 L18 | A1 L15 S5 L16 L7 S1 L6
sketch "Sketch4" plane through (0, 0, 2.54) normal (0, 0, 1) x (1, 0, 0)
  spline S0 degree 3 poles (0.2252, 51.1622) (0.8569, 51.1081) (2.2201, 51.0318) (4.1484, 51.014) (6.2204, 51.0558) (7.9821, 51.1377) (10.2866, 51.3027) (12.2007, 51.4858) (14.6529, 51.7811) (16.6505, 52.0715) (19.1637, 52.5051) (21.1754, 52.9097) (23.6629, 53.4906) (25.6198, 54.0171) (27.9963, 54.7565) (30.2893, 55.5796) (32.0054, 56.3339) (32.8267, 56.7373) knots 0.006523 0.006523 0.006523 0.006523 0.086155 0.165786 0.205602 0.285233 0.325048 0.40468 0.444495 0.524127 0.563942 0.643574 0.683389 0.76302 0.802836 0.882467 0.962099 0.962099 0.962099 0.962099 projected
  line L0 (32.8267, 56.7373) -> (50.5783, 38.8306) projected
  spline S1 degree 3 poles (50.5783, 38.8306) (50.4465, 38.5608) (50.1733, 37.9696) (49.8044, 37.11) (49.4181, 36.1732) (49.097, 35.3681) (48.6847, 34.3067) (48.3481, 33.4195) (47.9232, 32.2764) (47.5817, 31.3399) (47.1569, 30.154) (46.8201, 29.1975) (46.4065, 28.0022) (46.0827, 27.05) (45.6898, 25.8731) (45.3859, 24.945) (45.0215, 23.808) (44.743, 22.9189) (44.413, 21.8373) (44.164, 20.997) (43.8727, 19.98) (43.6558, 19.1935) (43.4055, 18.2442) (43.222, 17.5114) (43.0136, 16.627) (42.8635, 15.9434) (42.6963, 15.1155) (42.5786, 14.4726) (42.4248, 13.5316) (42.3005, 12.6171) (42.177, 11.4173) (42.1107, 10.5157) (42.0591, 9.5946) (42.031, 8.9681) (42.001, 8.1629) (41.9801, 7.4988) (41.9554, 6.6391) (41.9358, 5.9261) (41.9093, 5.0003) (41.8855, 4.2314) (41.8503, 3.2341) (41.8169, 2.4076) (41.7564, 1.1264) (41.6803, -0.2078) (41.5281, -2.293) (41.3467, -4.2245) (41.0555, -6.7073) (40.7699, -8.7362) (40.3501, -11.2957) (39.9673, -13.35) (39.4951, -15.6418) (39.1624, -17.1512) (38.8207, -18.6367) (38.5892, -19.6138) (38.2965, -20.8164) (38.0601, -21.7626) (37.7625, -22.9243) (37.5228, -23.8366) (37.2211, -24.9556) (36.978, -25.8339) (36.6708, -26.9118) (36.4221, -27.7589) (36.0426, -29.0096) (35.6529, -30.2362) (35.1065, -31.847) (34.6697, -33.0475) (34.2026, -34.2564) (33.8748, -35.0685) (33.4417, -36.0956) (33.0757, -36.9283) (32.5919, -37.9855) (32.1832, -38.845) (31.6443, -39.9374) (31.1906, -40.8259) (30.5951, -41.9538) (30.0963, -42.8694) (29.4455, -44.0283) (28.9036, -44.9657) (28.2014, -46.1464) (27.6207, -47.0964) (26.7244, -48.523) (25.7971, -49.9468) (24.5223, -51.8149) (23.5437, -53.1819) (22.5537, -54.5101) (21.889, -55.3744) (21.0547, -56.4247) (20.3854, -57.2394) (19.5483, -58.223) (18.8791, -58.9811) (18.0449, -59.8908) (17.3799, -60.5877) (16.5528, -61.4191) (15.8949, -62.0523) (15.0781, -62.804) (14.4294, -63.3735) (13.6245, -64.0468) (12.9855, -64.5551) (12.1926, -65.1544) (11.5627, -65.6061) (10.7799, -66.1387) (10.1567, -66.5407) (9.2248, -67.1119) (8.295, -67.6441) (6.8944, -68.3904) (5.6345, -69.015) (4.0198, -69.7969) (2.3545, -70.6081) (0.9495, -71.3557) (0.2252, -71.7733) knots 0.019866 0.019866 0.019866 0.019866 0.02999 0.040114 0.045176 0.0553 0.060362 0.070486 0.075548 0.085672 0.090734 0.100858 0.10592 0.116045 0.121107 0.131231 0.136293 0.146417 0.151479 0.161603 0.166665 0.176789 0.181851 0.191975 0.197037 0.207161 0.212223 0.222347 0.227409 0.242595 0.25272 0.267906 0.272968 0.283092 0.288154 0.298278 0.30334 0.313464 0.318526 0.32865 0.333712 0.343836 0.348898 0.364084 0.374208 0.394457 0.404581 0.424829 0.434953 0.455201 0.465325 0.480511 0.485573 0.495697 0.500759 0.510883 0.515945 0.52607 0.531132 0.541256 0.546318 0.556442 0.561504 0.57669 0.586814 0.602 0.607062 0.617186 0.622248 0.632372 0.637434 0.647558 0.65262 0.662745 0.667807 0.677931 0.682993 0.693117 0.698179 0.708303 0.713365 0.728551 0.738675 0.753861 0.758923 0.769047 0.774109 0.784233 0.789295 0.79942 0.804482 0.814606 0.819668 0.829792 0.834854 0.844978 0.85004 0.860164 0.865226 0.87535 0.880412 0.890536 0.895598 0.910784 0.920908 0.941157 0.951281 0.971529 0.991777 0.991777 0.991777 0.991777 projected
  spline S2 degree 3 poles (0.2252, -71.7733) (-0.4991, -71.3557) (-1.9041, -70.6081) (-3.5693, -69.7969) (-5.1841, -69.015) (-6.4439, -68.3904) (-7.8446, -67.6441) (-8.7744, -67.1119) (-9.7063, -66.5407) (-10.3294, -66.1387) (-11.1123, -65.6061) (-11.7422, -65.1544) (-12.5351, -64.5551) (-13.1741, -64.0468) (-13.9789, -63.3735) (-14.6277, -62.804) (-15.4445, -62.0523) (-16.1024, -61.4191) (-16.9294, -60.5877) (-17.5945, -59.8908) (-18.4287, -58.9811) (-19.0979, -58.223) (-19.9349, -57.2394) (-20.6043, -56.4247) (-21.4386, -55.3744) (-22.1033, -54.5101) (-23.0933, -53.1819) (-24.0719, -51.8149) (-25.3467, -49.9468) (-26.274, -48.523) (-27.1703, -47.0964) (-27.751, -46.1464) (-28.4532, -44.9657) (-28.9951, -44.0283) (-29.6459, -42.8694) (-30.1447, -41.9538) (-30.7402, -40.8259) (-31.1939, -39.9374) (-31.7327, -38.845) (-32.1414, -37.9855) (-32.6253, -36.9283) (-32.9913, -36.0956) (-33.4243, -35.0685) (-33.7522, -34.2564) (-34.2192, -33.0475) (-34.6561, -31.847) (-35.2025, -30.2362) (-35.5922, -29.0096) (-35.9717, -27.7589) (-36.2204, -26.9118) (-36.5275, -25.8339) (-36.7707, -24.9556) (-37.0724, -23.8366) (-37.312, -22.9243) (-37.6096, -21.7626) (-37.846, -20.8164) (-38.1388, -19.6138) (-38.3703, -18.6367) (-38.712, -17.1512) (-39.0446, -15.6418) (-39.5168, -13.35) (-39.8997, -11.2957) (-40.3195, -8.7362) (-40.6051, -6.7073) (-40.8963, -4.2245) (-41.0776, -2.293) (-41.2299, -0.2078) (-41.3059, 1.1264) (-41.3664, 2.4076) (-41.3998, 3.2341) (-41.435, 4.2314) (-41.4589, 5.0003) (-41.4854, 5.9261) (-41.505, 6.6391) (-41.5297, 7.4988) (-41.5505, 8.1629) (-41.5806, 8.9681) (-41.6087, 9.5946) (-41.6603, 10.5157) (-41.7265, 11.4173) (-41.8501, 12.6171) (-41.9744, 13.5316) (-42.1282, 14.4726) (-42.2459, 15.1155) (-42.4131, 15.9434) (-42.5631, 16.627) (-42.7716, 17.5114) (-42.955, 18.2442) (-43.2053, 19.1935) (-43.4222, 19.98) (-43.7136, 20.997) (-43.9626, 21.8373) (-44.2926, 22.9189) (-44.5711, 23.808) (-44.9355, 24.945) (-45.2394, 25.8731) (-45.6323, 27.05) (-45.956, 28.0022) (-46.3697, 29.1975) (-46.7064, 30.154) (-47.1313, 31.3399) (-47.4728, 32.2764) (-47.8977, 33.4195) (-48.2343, 34.3067) (-48.6465, 35.3681) (-48.9677, 36.1732) (-49.354, 37.11) (-49.7229, 37.9696) (-49.9961, 38.5608) (-50.1278, 38.8306) knots 0.019866 0.019866 0.019866 0.019866 0.040114 0.060362 0.070486 0.090734 0.100858 0.116045 0.121107 0.131231 0.136293 0.146417 0.151479 0.161603 0.166665 0.176789 0.181851 0.191975 0.197037 0.207161 0.212223 0.222347 0.227409 0.237533 0.242595 0.25272 0.257782 0.272968 0.283092 0.298278 0.30334 0.313464 0.318526 0.32865 0.333712 0.343836 0.348898 0.359022 0.364084 0.374208 0.37927 0.389395 0.394457 0.404581 0.409643 0.424829 0.434953 0.450139 0.455201 0.465325 0.470387 0.480511 0.485573 0.495697 0.500759 0.510883 0.515945 0.52607 0.531132 0.546318 0.556442 0.57669 0.586814 0.607062 0.617186 0.637434 0.647558 0.662745 0.667807 0.677931 0.682993 0.693117 0.698179 0.708303 0.713365 0.723489 0.728551 0.738675 0.743737 0.758923 0.769047 0.784233 0.789295 0.79942 0.804482 0.814606 0.819668 0.829792 0.834854 0.844978 0.85004 0.860164 0.865226 0.87535 0.880412 0.890536 0.895598 0.905722 0.910784 0.920908 0.92597 0.936095 0.941157 0.951281 0.956343 0.966467 0.971529 0.981653 0.991777 0.991777 0.991777 0.991777 projected
  line L1 (-50.1278, 38.8306) -> (-32.3763, 56.7373) projected
  spline S3 degree 3 poles (-32.3763, 56.7373) (-31.555, 56.3339) (-29.8389, 55.5796) (-27.5459, 54.7565) (-25.1694, 54.0171) (-23.2125, 53.4906) (-20.725, 52.9097) (-18.7132, 52.5051) (-16.2001, 52.0715) (-14.2024, 51.7811) (-11.7503, 51.4858) (-9.8362, 51.3027) (-7.5316, 51.1377) (-5.77, 51.0558) (-3.698, 51.014) (-1.7696, 51.0318) (-0.4065, 51.1081) (0.2252, 51.1622) knots 0.006523 0.006523 0.006523 0.006523 0.086155 0.165786 0.205602 0.285233 0.325048 0.40468 0.444495 0.524127 0.563942 0.643574 0.683389 0.76302 0.802836 0.882467 0.962099 0.962099 0.962099 0.962099 projected
  point P0 (0, 0)
extrude "Extrusion3" add sketch "Sketch4" along normal blind 1.27
sketch "Sketch5" plane through (0.2252, 1.113, 3.81) normal (0, 0, 1) x (1, 0, 0)
  arc A0 (18.4923, -14.9478) -> (14.1691, 23.9655) centre (0.467, 2.7465) ccw projected
  line L0 (14.4714, -22.164) -> (14.1691, 23.9655) projected
  line L1 (18.4923, -18.108) -> (14.4714, -22.164) projected
  line L2 (18.4923, -14.9478) -> (18.4923, -18.108) projected
  line L3 (19.0084, -7.1637) -> (19.0084, 10.2944) projected
  arc A1 (19.0084, -7.1637) -> (19.0084, 10.2944) centre (7.4469, 1.5654) ccw projected
  line L4 (10.9101, 20.4494) -> (10.9101, -3.2101) projected
  arc A2 (10.9101, 20.4494) -> (-2.245, 27.7127) centre (-0.7473, 14.8805) ccw projected
  line L5 (-2.245, 27.7127) -> (-2.245, -26.458) projected
  line L6 (2.036, 22.3033) -> (2.036, -5.8153) projected
  arc A3 (5.7582, 20.779) -> (2.036, 22.3033) centre (0.9724, 14.3993) ccw projected
  line L7 (5.7582, -1.4418) -> (5.7582, 20.779) projected
  arc A4 (2.036, -5.8153) -> (5.7582, -1.4418) centre (-1.7652, 1.1904) ccw projected
  arc A5 (5.7582, -9.2553) -> (10.9101, -3.2101) centre (2.6694, -1.4051) ccw projected
  line L8 (11.4659, -23.5658) -> (5.7582, -9.2553) projected
  line L9 (7.3581, -25.3269) -> (11.4659, -23.5658) projected
  line L10 (2.036, -14.2176) -> (7.3581, -25.3269) projected
  line L11 (2.036, -26.458) -> (2.036, -14.2176) projected
  line L12 (-2.245, -26.458) -> (2.036, -26.458) projected
  line L13 (-5.0408, -21.1435) -> (-5.0408, -25.988) projected
  arc A6 (-5.1396, 22.3033) -> (-5.0408, -21.1435) centre (0.4845, 0.5925) ccw projected
  arc A7 (-5.1396, 27.3992) -> (-5.0408, -25.988) centre (-0.2474, 0.7146) ccw projected
  line L14 (-5.1396, 27.3992) -> (-5.1396, 22.3033) projected
  arc A8 (-5.784, 20.779) -> (-13.2169, -14.2891) centre (1.3246, 0.9505) ccw projected
  line L15 (-5.784, -17.4837) -> (-5.784, 20.779) projected
  arc A9 (-9.8958, 12.1065) -> (-15.1944, 3.1301) centre (-2.7644, 1.8449) ccw projected
  line L16 (-9.8958, 12.1065) -> (-9.8958, 3.1301) projected
  line L17 (-9.8958, 3.1301) -> (-15.1944, 3.1301) projected
  line L18 (-15.1944, -1.4418) -> (-9.8958, -1.4418) projected
  line L19 (-9.8958, -1.4418) -> (-9.8958, -17.4837) projected
  arc A10 (-15.1944, -1.4418) -> (-10.7204, -9.6356) centre (-2.7006, 0.0616) ccw projected
  line L20 (-10.7204, -9.6356) -> (-13.2169, -14.2891) projected
  line L21 (-9.8958, -17.4837) -> (-5.784, -17.4837) projected
  point P0 (-0.2252, -1.113)
extrude "Extrusion4" add sketch "Sketch5" along normal blind 1.27
sketch "Sketch7" plane through (0, 0, 0) normal (0, 0, -1) x (-1, 0, 0)
  line L0 (-0.2252, 52.8739) -> (-0.2252, 61.0122) construction
  arc A0 (7.4224, 52.8006) -> (-7.8452, 52.4981) centre (-0.2252, 53.3453) ccw
  line L1 (-0.2252, 53.3453) -> (-7.8452, 52.4981) construction
  arc A1 (-7.8452, 52.4981) -> (7.4224, 52.8006) centre (-0.4682, 65.6116) ccw
  line L2 (-0.2252, 53.3453) -> (-0.2252, 61.0122) construction
  circle A2 centre (-0.2252, 57.1787) radius 2.54
  point P0 (0, 0)
  dimension "d44" = 7.62
  dimension "d45" = 5.08
  constraints: 6 end point, 5 point on circle, 3 centre point, 2 vertical, 1 coincident, 1 midpoint, 1 point on line
  measures "d44" horizontal distance of L1.start L1.end
  measures "d45" diameter of A2
extrude "Extrusion5" add sketch "Sketch7" against normal blind 1.27
body "Solid1"
